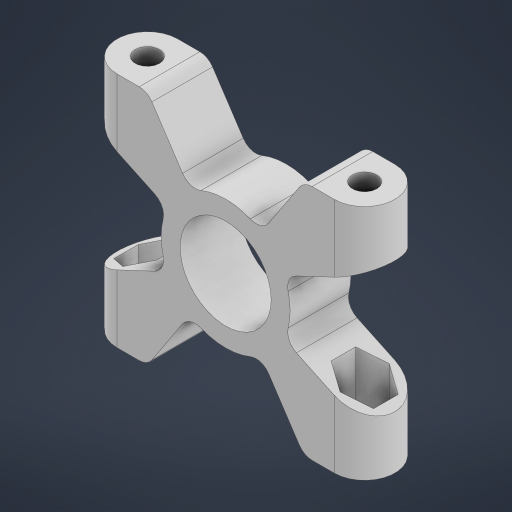
# Autodesk Inventor part: Center_Bracket
Saved by Autodesk Inventor 2023 (Build 270158000, 158)
## iProperties
Created: 2023-08-25
Part Number: Center_Bracket
Material: Generic
Document SubType Name: Modeling
Designer: Izack Waczko
Density: 1 g/cm^3
Appearance: Default
Author: Izack Waczko
Autodesk Inventor part; units mm, degrees
ref_plane "YZ Plane" through (0, 0, 0) normal (1, 0, 0) x (0, 1, 0)
ref_plane "XZ Plane" through (0, 0, 0) normal (0, 1, 0) x (-1, 0, 0)
ref_plane "XY Plane" through (0, 0, 0) normal (0, 0, 1) x (1, 0, 0)
sketch "Sketch1" plane through (0, 0, 0) normal (0, 1, 0) x (-1, 0, 0)
  line L0 (0, 0) -> (28.638, 0) construction
  circle A0 centre (28.638, 0) radius 1.6
  circle A1 centre (0, 0) radius 1.6
  circle A2 centre (28.638, 0) radius 4
  circle A3 centre (0, 0) radius 4
  line L1 (28.638, 4) -> (0, 4)
  line L2 (28.638, -4) -> (0, -4)
  dimension "d0" = 28.638
  dimension "d1" = 3.2
  dimension "d2" = 3.2
  dimension "d3" = 8
  dimension "d4" = 8
  constraints: 6 end point, 4 centre point, 4 coincident, 4 point on circle, 2 tangent, 1 horizontal
  measures "d0" distance of L0.start L0.end
  measures "d1" diameter of A0
  measures "d2" diameter of A1
  measures "d3" diameter of A2
  measures "d4" diameter of A3
extrude "Extrusion1" add sketch "Sketch1" along normal blind 31.25
sketch "Sketch2" plane through (-28.638, 0, 4) normal (0, 0, 1) x (1, 0, 0)
  line L0 (0, 31.25) -> (28.638, 31.25) construction
  line L1 (14.319, 31.25) -> (14.319, 0) construction
  line L2 (-4, 0) -> (-4, 31.25) construction
  line L3 (-4, 15.625) -> (32.638, 15.625) construction
  line L4 (32.638, 0) -> (32.638, 31.25) construction
  circle A0 centre (14.319, 15.625) radius 6
  line L5 (-4, 31.25) -> (-4, 24.25)
  line L6 (-4, 24.25) -> (4, 24.25) construction
  line L7 (1.6, 31.25) -> (1.6, 0) projected
  line L8 (4, 24.25) -> (4, 31.25) construction
  line L9 (4, 31.25) -> (9.6348, 22.7178)
  line L10 (-4, 24.25) -> (6.6287, 19.2458)
  line L11 (32.638, 24.25) -> (24.638, 24.25) construction
  line L12 (24.638, 24.25) -> (24.638, 31.25) construction
  line L13 (24.638, 31.25) -> (19.0032, 22.7178)
  line L14 (32.638, 24.25) -> (22.0093, 19.2458)
  line L15 (-4, 31.25) -> (4, 31.25)
  line L16 (32.638, 31.25) -> (28.638, 31.25) projected
  line L17 (24.638, 31.25) -> (32.638, 31.25)
  line L18 (32.638, 31.25) -> (32.638, 24.25)
  line L19 (0, 0) -> (28.638, 0) construction
  line L20 (-4, 0) -> (-4, 7)
  line L21 (4, 0) -> (9.6348, 8.5322)
  line L22 (-4, 7) -> (6.6287, 12.0042)
  line L23 (32.638, 7) -> (22.0093, 12.0042)
  line L24 (24.638, 0) -> (19.0032, 8.5322)
  line L25 (-4, 0) -> (4, 0)
  line L26 (32.638, 0) -> (28.638, 0)
  line L27 (24.638, 0) -> (32.638, 0)
  line L28 (32.638, 7) -> (32.638, 0)
  line L29 (32.638, 0) -> (24.638, 0)
  line L30 (0, 0) -> (28.638, 0) projected
  line L31 (0, 0) -> (-4, 0) projected
  line L32 (4, 0) -> (-4, 0)
  line L33 (-4, 0) -> (-4, 7)
  line L34 (4, 31.25) -> (24.638, 31.25)
  line L35 (32.638, 24.25) -> (32.638, 6.9357)
  line L36 (24.638, 0) -> (4, 0)
  line L37 (-4, 7) -> (-4, 24.25)
  circle A1 centre (14.319, 15.625) radius 8.5
  point P0 (8.8906, 13.0692)
  point P1 (11.0125, 10.6183)
  point P2 (17.6255, 10.6183)
  point P3 (19.7474, 13.0692)
  point P4 (17.6255, 10.6183)
  point P5 (11.0125, 10.6183)
  point P6 (19.7474, 13.0692)
  point P7 (8.8906, 13.0692)
  dimension "d12" = 17
  dimension "d7" = 12
  dimension "d8" = 7
  dimension "d9" = 8
  constraints: 62 end point, 9 symmetric about line, 6 collinear, 4 midpoint, 4 point on line, 3 perpendicular, 2 horizontal, 1 centre point, 1 coincident, 1 vertical, 10 other
  measures "d7" diameter of A0
  measures "d8" distance of L2.end L5.end
  measures "d9" distance of L5.end L6.end
extrude "Extrusion2" cut sketch "Sketch2" against normal through all contours A0 | L10 L7 L22 L37 | L10 A1 L22 L7 | L34 L13 A1 L9 | L21 A1 L24 L30 | L14 L35 L23 A1
ref_plane "Work Plane1" through (0, 15.625, 0) normal (0, 1, 0) x (1, 0, 0)
sketch "Sketch3" plane through (0, 15.625, 0) normal (0, 1, 0) x (1, 0, 0)
  circle A0 centre (-28.638, 0) radius 1.6 projected
  circle A1 centre (-28.638, 0) radius 2.8 construction
  circle A2 centre (0, 0) radius 2.8 construction
  line L0 (-25.838, -1.6166) -> (-28.638, -3.2332)
  line L1 (-28.638, -3.2332) -> (-31.438, -1.6166)
  line L2 (-31.438, -1.6166) -> (-31.438, 1.6166)
  line L3 (-31.438, 1.6166) -> (-28.638, 3.2332)
  line L4 (-28.638, 3.2332) -> (-25.838, 1.6166)
  line L5 (-25.838, 1.6166) -> (-25.838, -1.6166)
  line L6 (2.8, -1.6166) -> (0, -3.2332)
  line L7 (0, -3.2332) -> (-2.8, -1.6166)
  line L8 (-2.8, -1.6166) -> (-2.8, 1.6166)
  line L9 (-2.8, 1.6166) -> (0, 3.2332)
  line L10 (0, 3.2332) -> (2.8, 1.6166)
  line L11 (2.8, 1.6166) -> (2.8, -1.6166)
  point P0 (-25.838, 0)
  point P1 (2.8, 0)
  dimension "d13" = 5.6
  dimension "d14" = 5.6
  constraints: 24 end point, 4 coincident, 2 horizontal alignment, 2 midpoint, 30 other
extrude "Extrusion3" cut sketch "Sketch3" along normal mid plane 25.25 contours A0 | L0 L1 L2 L3 L4 L5 | L6 L7 L8 L9 L10 L11
fillet "Fillet1" radius 2 12 edges at (-24.638, 31.25, 0) (-19.0032, 22.7178, 0) (-9.6348, 22.7178, 0) (-4, 31.25, 0) (-6.6287, 19.2458, 0) (-6.6287, 12.0042, 0) (-9.6348, 8.5322, 0) (-4, 0, 0) (-24.638, 0, 0) (-19.0032, 8.5322, 0) (-22.0093, 12.0042, 0) (-22.0093, 19.2458, 0)
body "Solid1"
